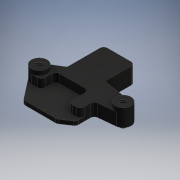
# Autodesk Inventor part: EPS_RegulatorHeatsink-B
Saved by Autodesk Inventor 2018 (Build 220112000, 112)
## iProperties
Created: 2018-09-29
Part Number: EPS_RegulatorHeatsink-B
Material: Aluminum 6061
Document SubType Name: Modeling
Designer: Bradley
Density: 2.7 g/cm^3
Appearance: Anodized - Dark Gray
Mass: 1.86381 g
Surface Area: 8.94347 cm^2
Volume: 0.6903 cm^3
Author: Bradley
Autodesk Inventor part; units mm, degrees
ref_plane "YZ Plane" through (0, 0, 0) normal (1, 0, 0) x (0, 1, 0)
ref_plane "XZ Plane" through (0, 0, 0) normal (0, 1, 0) x (-1, 0, 0)
ref_plane "XY Plane" through (0, 0, 0) normal (0, 0, 1) x (1, 0, 0)
sketch "Sketch1" plane through (0, 0, 0) normal (0, 0, 1) x (1, 0, 0)
  circle A0 centre (0, 0) radius 2
  circle A1 centre (19, 2.5) radius 2
  dimension "d0" = 19
  dimension "d2" = 2.5
  dimension "d3" = 4
  constraints: 2 centre point, 1 coincident, 1 equal radius
  measures "d0" horizontal distance of A0.centre A1.centre
  measures "d2" vertical distance of A0.centre A1.centre
  measures "d3" diameter of A0
extrude "Extrusion1" add sketch "Sketch1" along normal mid plane 3.4
sketch "Sketch2" plane through (0, 0, -1.7) normal (0, 0, -1) x (-1, 0, 0)
  circle A0 centre (-19, 2.5) radius 2 projected
  circle A1 centre (0, 0) radius 2 projected
  line L0 (-2.95, 1.25) -> (-10.45, 1.25) construction
  line L1 (-10.45, 1.25) -> (-10.45, -6.25) construction
  line L2 (-10.45, -6.25) -> (-2.95, -6.25) construction
  line L3 (-2.95, -6.25) -> (-2.95, 1.25) construction
  line L4 (-9.875, 5.65) -> (-6.725, 5.65) construction
  line L5 (-6.725, 5.65) -> (-6.725, 2.5) construction
  line L6 (-6.725, 2.5) -> (-9.875, 2.5) construction
  line L7 (-9.875, 2.5) -> (-9.875, 5.65) construction
  line L8 (-13.55, -1.3) -> (-11.65, -1.3) construction
  line L9 (-11.65, -1.3) -> (-11.65, -4.3) construction
  line L10 (-11.65, -4.3) -> (-13.55, -4.3) construction
  line L11 (-13.55, -4.3) -> (-13.55, -1.3) construction
  line L12 (-11, -6.5) -> (-2.5, -6.5)
  line L13 (-2.5, -6.5) -> (1.5819, -1.2238)
  circle A2 centre (0, 0) radius 2 projected
  line L14 (1.041, 1.7077) -> (-6, 6)
  line L15 (-6, 6) -> (-10.5, 6)
  line L16 (-10.5, 6) -> (-19.3409, 4.4707)
  circle A3 centre (-19, 2.5) radius 2 projected
  line L17 (-19.1952, 0.5096) -> (-14, 0)
  line L18 (-14, 0) -> (-14, -4.5)
  line L19 (-14, -4.5) -> (-11, -6.5)
  circle A4 centre (-19, 2.5) radius 2 projected
  line L20 (-3, 13.5) -> (-11, 13.5)
  line L21 (-3, 13.5) -> (-3, 4.1712)
  line L22 (-11, 13.5) -> (-11, 5.9135)
  dimension "d15" = 7.5
  dimension "d16" = 1.25
  dimension "d17" = 2.95
  dimension "d18" = 6.725
  dimension "d19" = 3.15
  dimension "d20" = 2.5
  dimension "d21" = 1.9
  dimension "d22" = 3
  dimension "d23" = 11.65
  dimension "d24" = 1.3
  dimension "d25" = 6
  dimension "d26" = 6.5
  dimension "d27" = 2.5
  dimension "d28" = 6
  dimension "d29" = 8.5
  dimension "d30" = 5
  dimension "d31" = 2
  dimension "d32" = 11
  dimension "d33" = 2.5
  dimension "d42" = 7.5
  dimension "d43" = 8
  dimension "d44" = 3
  constraints: 46 end point, 8 parallel, 6 perpendicular, 5 horizontal, 4 point on circle, 4 tangent, 2 point on line, 1 vertical
  measures "d15" distance of L2.end L1.end
  measures "d16" distance from line of L0 point (0, 0)
  measures "d17" distance from line of L3 point (0, 0)
  measures "d18" distance from line of point (0, 0) L5
  measures "d19" distance of L4.start L4.end
  measures "d20" distance from line of point (0, 0) L6
  measures "d21" distance of L8.start L8.end
  measures "d22" distance of L10.end L8.start
  measures "d23" distance from line of point (0, 0) L9
  measures "d24" distance from line of L8 point (0, 0)
  measures "d25" distance from line of point (0, 0) L15
  measures "d26" distance from line of L12 point (0, 0)
  measures "d27" horizontal distance of L12.end point (0, 0)
  measures "d28" horizontal distance of point (0, 0) L14.end
  measures "d29" horizontal distance of L15.end A0.centre
  measures "d30" distance from line of L18 A0.centre
  measures "d31" distance from line of L18.end L12
  measures "d32" horizontal distance of A1.centre L12.start
  measures "d33" vertical distance of L17.end A0.centre
  measures "d42" distance between parallel lines of L15 L20
  measures "d43" distance of L20.start L20.end
  measures "d44" distance from line of point (0, 0) L21
extrude "Extrusion2" add sketch "Sketch2" along normal blind 1
sketch "Sketch3" plane through (0, 0, 1.7) normal (0, 0, 1) x (1, 0, 0)
  circle A0 centre (0, 0) radius 2 projected
  circle A1 centre (19, 2.5) radius 2 projected
hole "Hole1" at (0, 0, 1.7) at (19, 2.5, 1.7) direction (0, 0, -1) diameter 1.567 end through all thread size "M2x0.4" class "6H" standard "ANSI Metric M Profile"
fillet "Fillet1" radius 1 4 edges at (14, 0, -2.2) (14, -4.5, -2.2) (2.5, -6.5, -2.2) (11, -6.5, -2.2)
sketch "Sketch4" plane through (0, 0, -1.7) normal (0, 0, 1) x (1, 0, 0)
  line L0 (-1.041, 1.7077) -> (3, 4.1712) projected
  arc A0 (-1.5819, -1.2238) -> (-1.041, 1.7077) centre (0, 0) ccw projected
  line L1 (2.1997, -6.1119) -> (-1.5819, -1.2238) projected
  arc A1 (2.1997, -6.1119) -> (2.9907, -6.5) centre (2.9907, -5.5) ccw projected
  line L2 (10.6972, -6.5) -> (2.9907, -6.5) projected
  arc A2 (10.6972, -6.5) -> (11.2519, -6.3321) centre (10.6972, -5.5) ccw projected
  line L3 (13.5547, -4.7969) -> (11.2519, -6.3321) projected
  arc A3 (13.5547, -4.7969) -> (14, -3.9648) centre (13, -3.9648) ccw projected
  line L4 (14, -0.9067) -> (14, -3.9648) projected
  arc A4 (14.9024, 0.0885) -> (14, -0.9067) centre (15, -0.9067) ccw projected
  line L5 (19.1952, 0.5096) -> (14.9024, 0.0885) projected
  arc A5 (19.3409, 4.4707) -> (19.1952, 0.5096) centre (19, 2.5) ccw projected
  line L6 (11, 5.9135) -> (19.3409, 4.4707) projected
  line L7 (2.95, 1.25) -> (10.45, 1.25) construction
  line L8 (2.95, -6.25) -> (2.95, 1.25) construction
  line L9 (10.45, 1.25) -> (10.45, -6.25) construction
  line L10 (10.45, -6.25) -> (2.95, -6.25) construction
  circle A6 centre (0, 0) radius 2 projected
  line L11 (0, -2) -> (2.5, -2)
  line L12 (2.5, -2) -> (2.5, 1.75)
  line L13 (2.5, 1.75) -> (11, 1.75)
  line L14 (11, 1.75) -> (11, -3.5)
  line L15 (11, -3.5) -> (14, -3.5)
  line L16 (11, 13.5) -> (11, 5.9135) projected
  line L17 (3, 13.5) -> (11, 13.5) projected
  line L18 (3, 4.1712) -> (3, 13.5) projected
  dimension "d35" = 2.5
  dimension "d36" = 1.75
  dimension "d37" = 11
  dimension "d38" = 3.5
  constraints: 10 end point, 3 perpendicular, 1 horizontal, 1 parallel, 1 point on circle, 1 point on line, 1 tangent
  measures "d35" distance from line of L12 point (0, 0)
  measures "d36" distance from line of A0.centre L13
  measures "d37" distance from line of L14 point (0, 0)
  measures "d38" distance from line of L15 point (0, 0)
extrude "Extrusion3" add sketch "Sketch4" along normal blind 2.215 contours L0 L18 L17 L16 L6 A5 L5 A4 L4 L15 L14 L13 L12 L11 A0
fillet "Fillet2" radius 1 7 edges at (2.5, -2, -0.5925) (2.5, 1.75, -0.5925) (11, 1.75, -0.5925) (11, -3.5, -0.5925) (14, -3.5, -0.5925) (11, 13.5, -1.0925) (3, 13.5, -1.0925)
sketch "Sketch5" plane through (0, 0, -2.7) normal (0, 0, -1) x (-1, 0, 0)
  arc A0 (-11.2519, -6.3321) -> (-10.6972, -6.5) centre (-10.6972, -5.5) ccw projected
  line L0 (-10.6972, -6.5) -> (-2.9907, -6.5) projected
  arc A1 (-2.9907, -6.5) -> (-2.1997, -6.1119) centre (-2.9907, -5.5) ccw projected
  line L1 (-2.1997, -6.1119) -> (1.5819, -1.2238) projected
  arc A2 (1.5819, -1.2238) -> (1.041, 1.7077) centre (0, 0) ccw projected
  line L2 (1.041, 1.7077) -> (-3, 4.1712) projected
  line L3 (-3, 4.1712) -> (-3, 12.5) projected
  line L4 (-4, 13.5) -> (-10, 13.5) projected
  line L5 (-11, 12.5) -> (-11, 5.9135) projected
  line L6 (-11, 5.9135) -> (-19.3409, 4.4707) projected
  arc A3 (-19.3409, 4.4707) -> (-19.1952, 0.5096) centre (-19, 2.5) ccw projected
  line L7 (-19.1952, 0.5096) -> (-14.9024, 0.0885) projected
  arc A4 (-14, -0.9067) -> (-14.9024, 0.0885) centre (-15, -0.9067) ccw projected
  line L8 (-14, -0.9067) -> (-14, -3.9648) projected
  arc A5 (-14, -3.9648) -> (-13.5547, -4.7969) centre (-13, -3.9648) ccw projected
  line L9 (-13.5547, -4.7969) -> (-11.2519, -6.3321) projected
  circle A6 centre (-19, 2.5) radius 0.7835 projected
  circle A7 centre (0, 0) radius 0.7835 projected
  line L10 (-11, 7.5) -> (-3, 7.5)
  arc A8 (-3, 12.5) -> (-4, 13.5) centre (-4, 12.5) ccw projected
  arc A9 (-10, 13.5) -> (-11, 12.5) centre (-10, 12.5) ccw projected
  line L11 (-3, 4.1712) -> (-3, 12.5) projected
  dimension "d45" = 6
  constraints: 2 end point, 2 point on line
  measures "d45" distance between parallel lines of L4 L10
extrude "Extrusion4" add sketch "Sketch5" along normal blind 1 contours L10 L5 A9 L4 A8 L3 | A6 | A7
chamfer "Chamfer1" distance 1 angle 45 1 edges at (7, 7.5, -2.7)
sketch "Sketch6" plane through (3, 13.5, 0.515) normal (0, 1, 0) x (1, 0, 0)
  line L0 (7, 0) -> (1, 0) projected
  line L1 (1, 4.215) -> (7, 0) construction
  line L2 (1, 0) -> (1, 4.215) projected
  line L3 (7, 4.215) -> (7, 0) projected
  line L4 (1, 4.215) -> (7, 4.215) projected
  point P0 (-3, 0.515)
  point P1 (4, 2.1075)
  constraints: 2 end point, 1 midpoint
hole "Hole2" at (7, 13.5, -1.5925) direction (0, -1, 0) diameter 1.567 depth 4 tip angle 118 thread size "M2x0.4" class "6H" standard "ANSI Metric M Profile"
body "Solid1"
